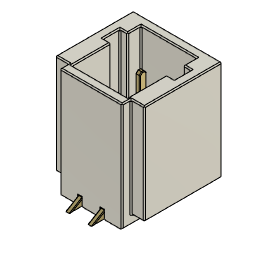
SH1.0mm_2P_立贴 (Autodesk Fusion 360 design; units mm, degrees)
Autodesk Fusion 360 part; units mm, degrees
sketch "草图1" plane through (0, 0, 0) normal (0, 0, 1) x (1, 0, 0) in component "Component'"
  line L0 (0, 0) -> (4, 0)
  line L1 (4, 0) -> (4, 3.9)
  line L2 (4, 3.9) -> (0, 3.9)
  line L3 (0, 3.9) -> (0, 0)
  dimension "d1" = 4
  dimension "d2" = 3.9
  constraint horizontal L0
  constraint vertical L1
  constraint horizontal L2
  constraint vertical L3
  constraint coincident L0.start L3.end
  measures "d1" distance of L0.start L0.end
  measures "d2" distance of L0.end L1.end
extrude "拉伸1" add sketch "草图1" along normal blind 4.9 makes body 1 in component "Component'"
sketch "草图2" plane through (0, 0, 4.9) normal (0, 0, 1) x (-1, 0, 0) in component "Component'"
  line L0 (0, -3.9) -> (0, 0)
  line L1 (0, 0) -> (-4, 0)
  line L2 (-4, 0) -> (-4, -3.9)
  line L3 (-4, -3.9) -> (0, -3.9)
  line L4 (-0.75, -0.4) -> (-3.25, -0.4)
  line L5 (-3.25, -0.4) -> (-3.25, -3.5)
  line L6 (-3.25, -3.5) -> (-0.75, -3.5)
  line L7 (-0.75, -3.5) -> (-0.75, -0.4)
  line L8 (-0.4, -2.9) -> (-3.6, -2.9)
  line L9 (-3.6, -2.9) -> (-3.6, -2.15)
  line L10 (-3.6, -2.15) -> (-0.4, -2.15)
  line L11 (-0.4, -2.15) -> (-0.4, -2.9)
  dimension "d5" = 2.5
  dimension "d6" = 0.75
  dimension "d7" = 0.4
  dimension "d8" = 0.4
  dimension "d9" = 3.2
  dimension "d10" = 0.4
  dimension "d11" = 1
  dimension "d12" = 0.75
  constraint horizontal L4
  constraint vertical L5
  constraint horizontal L6
  constraint vertical L7
  constraint horizontal L8
  constraint vertical L9
  constraint horizontal L10
  constraint vertical L11
  measures "d5" distance of L4.start L4.end
  measures "d6" distance of L2 L5
  measures "d7" distance of L3 L6
  measures "d8" distance of L1 L4
  measures "d9" distance of L9.end L10.end
  measures "d10" distance of L2 L9
  measures "d11" distance of L3 L8
  measures "d12" distance of L8.start L10.end
extrude "拉伸2" cut sketch "草图2" against normal blind 4 contours L4 L5 L7 L10 | L7 L8 L10 L11 | L5 L7 L8 L10 | L5 L8 L9 L10 | L5 L6 L7 L8 bodies 1 in component "Component'"
sketch "草图3" plane through (0, 0, 4.9) normal (0, 0, 1) x (-1, 0, 0) in component "Component'"
  line L0 (-3.25, -0.4) -> (-0.75, -0.4)
  line L1 (-0.75, -0.4) -> (-0.75, -2.15)
  line L2 (-0.75, -2.15) -> (-0.4, -2.15)
  line L3 (-0.4, -2.15) -> (-0.4, -2.9)
  line L4 (-0.4, -2.9) -> (-0.75, -2.9)
  line L5 (-0.75, -2.9) -> (-0.75, -3.5)
  line L6 (-0.75, -3.5) -> (-3.25, -3.5)
  line L7 (-3.25, -3.5) -> (-3.25, -2.9)
  line L8 (-3.25, -2.9) -> (-3.6, -2.9)
  line L9 (-3.6, -2.9) -> (-3.6, -2.15)
  line L10 (-3.6, -2.15) -> (-3.25, -2.15)
  line L11 (-3.25, -2.15) -> (-3.25, -0.4)
  line L12 (0, -3.9) -> (0, 0)
  line L13 (0, 0) -> (-4, 0)
  line L14 (-4, 0) -> (-4, -3.9)
  line L15 (-4, -3.9) -> (0, -3.9)
  line L16 (0, 0) -> (-0.6, 0)
  line L17 (-0.6, 0) -> (-0.6, -0.4)
  line L18 (-0.6, -0.4) -> (0, -0.4)
  line L19 (0, -0.4) -> (0, 0)
  line L20 (-4, 0) -> (-3.4, 0)
  line L21 (-3.4, 0) -> (-3.4, -0.4)
  line L22 (-3.4, -0.4) -> (-4, -0.4)
  line L23 (-4, -0.4) -> (-4, 0)
  dimension "d15" = 0.4
  dimension "d16" = 0.6
  dimension "d17" = 0.6
  dimension "d18" = 0.4
  constraint horizontal L16
  constraint vertical L17
  constraint horizontal L18
  constraint vertical L19
  constraint coincident L12.end L13.start
  constraint horizontal L20
  constraint vertical L21
  constraint horizontal L22
  constraint vertical L23
  constraint coincident L13.end L14.start
  measures "d15" distance of L16.end L17.end
  measures "d16" distance of L17.end L18.end
  measures "d17" distance of L21.end L22.end
  measures "d18" distance of L20.end L21.end
extrude "拉伸3" cut sketch "草图3" against normal up to surface (4.9 mm away) contours L12 L13 L16 L17 L18 L19 | L13 L14 L20 L21 L22 L23 bodies 1 in component "Component'"
sketch "草图4" plane through (0, 0, 0) normal (0, 0, -1) x (1, 0, 0) in component "Component'"
  line L0 (0.6, 0) -> (1.4, 0)
  line L1 (1.4, 0) -> (1.4, -3.9)
  line L2 (1.4, -3.9) -> (0.6, -3.9)
  line L3 (0.6, -3.9) -> (0.6, 0)
  line L4 (1.6, 0) -> (2.4, 0)
  line L5 (2.4, 0) -> (2.4, -3.9)
  line L6 (2.4, -3.9) -> (1.6, -3.9)
  line L7 (1.6, -3.9) -> (1.6, 0)
  line L8 (3.4, 0) -> (2.6, 0)
  line L9 (2.6, 0) -> (2.6, -3.9)
  line L10 (2.6, -3.9) -> (3.4, -3.9)
  line L11 (3.4, -3.9) -> (3.4, 0)
  line L12 (0, -3.9) -> (4, -3.9)
  line L13 (4, -3.9) -> (4, -3.5)
  line L14 (4, -3.5) -> (0, -3.5)
  line L15 (0, -3.5) -> (0, -3.9)
  line L16 (0, -3.5) -> (0, -0.4)
  line L17 (0, -0.4) -> (0.6, -0.4)
  line L18 (1.4, 0) -> (2.6, 0)
  line L19 (4, -3.5) -> (4, -0.4)
  line L20 (4, -0.4) -> (3.4, -0.4)
  point P0 (3.4, 0)
  dimension "d27" = 0.8
  dimension "d28" = 0.2
  dimension "d29" = 0.2
  dimension "d30" = 0.8
  dimension "d31" = 0.8
  dimension "d32" = 0.4
  constraint horizontal L0
  constraint vertical L1
  constraint horizontal L2
  constraint vertical L3
  constraint horizontal L4
  constraint vertical L5
  constraint horizontal L6
  constraint vertical L7
  constraint horizontal L8
  constraint vertical L9
  constraint horizontal L10
  constraint vertical L11
  constraint coincident P0 L8.start
  constraint horizontal L12
  constraint vertical L13
  constraint horizontal L14
  constraint vertical L15
  constraint perpendicular L14 L16
  constraint coincident L3 L17.end
  constraint perpendicular L3 L17
  constraint perpendicular L9 L18
  constraint perpendicular L14 L19
  constraint coincident L11 L20.end
  constraint perpendicular L11 L20
  measures "d27" distance of L4.start L4.end
  measures "d28" distance of L5 L9
  measures "d29" distance of L1 L7
  measures "d30" distance of P0 L8.end
  measures "d31" distance of L0.start L0.end
  measures "d32" distance of L12.end L13.end
extrude "拉伸5" cut sketch "草图4" against normal blind 0.4 contours L1 L7 L14 L18 | L3 L14 L16 L17 | L1 L7 L12 L14 | L1 L2 L3 L12 L14 | L3 L12 L14 L15 | L5 L6 L7 L12 L14 | L5 L9 L14 L18 | L5 L9 L12 L14 | L9 L10 L11 L12 L14 | L11 L12 L13 L14 | L11 L14 L19 L20 bodies 1 in component "Component'"
sketch "草图6" plane through (0, 0, 0.4) normal (0, 0, -1) x (1, 0, 0) in component "Component'"
  line L0 (0, -0.4) -> (0, -3.9)
  line L1 (0, -3.9) -> (4, -3.9)
  line L2 (4, -3.9) -> (4, -0.4)
  line L3 (4, -0.4) -> (3.4, -0.4)
  line L4 (3.4, -0.4) -> (3.4, -3.5)
  line L5 (3.4, -3.5) -> (2.6, -3.5)
  line L6 (2.6, -3.5) -> (2.6, 0)
  line L7 (2.6, 0) -> (2.4, 0)
  line L8 (2.4, 0) -> (2.4, -3.5)
  line L9 (2.4, -3.5) -> (1.6, -3.5)
  line L10 (1.6, -3.5) -> (1.6, 0)
  line L11 (1.6, 0) -> (1.4, 0)
  line L12 (1.4, 0) -> (1.4, -3.5)
  line L13 (1.4, -3.5) -> (0.6, -3.5)
  line L14 (0.6, -3.5) -> (0.6, -0.4)
  line L15 (0.6, -0.4) -> (0, -0.4)
  line L16 (1.4, -2.6) -> (1.6, -2.6)
  line L17 (1.6, -2.6) -> (1.6, -2.9)
  line L18 (1.6, -2.9) -> (1.4, -2.9)
  line L19 (1.4, -2.9) -> (1.4, -2.6)
  line L20 (2.4, -2.6) -> (2.6, -2.6)
  line L21 (2.6, -2.6) -> (2.6, -2.9)
  line L22 (2.6, -2.9) -> (2.4, -2.9)
  line L23 (2.4, -2.9) -> (2.4, -2.6)
  dimension "d35" = 0.3
  dimension "d36" = 1
  constraint horizontal L16
  constraint vertical L17
  constraint horizontal L18
  constraint vertical L19
  constraint coincident L10 L17.end
  constraint coincident L12 L16.start
  constraint horizontal L20
  constraint vertical L21
  constraint horizontal L22
  constraint vertical L23
  constraint coincident L6 L21.end
  constraint coincident L8 L20.start
  constraint collinear L18 L22
  constraint collinear L16 L20
  measures "d35" distance of L16.start L18.end
  measures "d36" distance of L1 L18
extrude "拉伸6" cut sketch "草图6" against normal up to surface (0.5 mm away) contours L10 L12 L16 L17 L18 L19 | L6 L8 L20 L21 L22 L23 bodies 1 in component "Component'"
sketch "草图1 (2)" plane through (1.4, 0, 0) normal (1, 0, 0) x (0, 1, 0) in component "Component''"
  line L0 (0, 0) -> (3.5, 0)
  line L1 (3.5, 0) -> (3.5, 0.4)
  line L2 (3.5, 0.4) -> (2.9, 0.4)
  line L3 (2.9, 0.4) -> (2.9, 0.9)
  line L4 (2.9, 0.9) -> (2.6, 0.9)
  line L5 (2.6, 0.9) -> (2.6, 0.4)
  line L6 (2.6, 0.4) -> (0, 0.4)
  line L7 (0, 0.4) -> (0, 0)
  line L8 (2.9, 0.4) -> (2.9, 3.9)
  line L9 (2.9, 3.9) -> (2.6, 3.9)
  line L10 (2.6, 3.9) -> (2.6, 0.4)
  line L11 (0.398, 0.4) -> (0.0284, 0.3471)
  line L12 (0.0284, 0.3471) -> (-0.55, 0)
  line L13 (-0.55, 0) -> (2.9, 0)
  line L14 (2.9, 0.4) -> (2.9, 0)
  line L15 (0, 0) -> (0, 4.9)
  dimension "d39" = 3.5
  dimension "d41" = 0.55
  constraint coincident L2.end L3.start
  constraint perpendicular L4 L8
  constraint perpendicular L8 L9
  constraint coincident L5.end L6.start
  constraint coincident L6 L11.start
  constraint coincident L0 L13.end
  constraint perpendicular L7 L13
  constraint vertical L14
  measures "d39" distance of L2.end L8.end
  measures "d41" distance of L12.end L15
extrude "拉伸1'" add sketch "草图1 (2)" along normal blind 0.2 separate body contours L0 L3 L4 L5 L6 L7 L8 L10 L11 L12 L13 L14 L15 | L7 L12 L13 L15 | L4 L8 L9 L10 makes body 2 in component "Component''"
chamfer "倒角1" distance 0.1 angle 45 2 edges at (1.5, 2.6, 3.9) (1.5, 2.9, 3.9) on bodies 2 in component "Component''"
fillet "圆角1" radius 0.25 1 edges at (1.5, 2.9, 0) on bodies 2 in component "Component''"
fillet "圆角2" radius 0.03 2 faces at (1.6, 0.8327, 0.1333) (1.4, 0.8327, 0.1333) on bodies 2 in component "Component''"
pattern_linear "R-阵列1" count 2 spacing 1 along (1, 0, 0) of bodies 2 makes body 3 in component "Component''"
chamfer "倒角1'" distance 0.05 angle 45 1 faces at (0.3333, 0.9833, 4.9) on bodies 1 in component "Component'"
chamfer "倒角2" distance 0.05 angle 45 31 edges at (0, 3.9, 2.625) (0, 0.4, 2.625) (0.6, 0.4, 2.625) (0.6, 0, 2.425) (3.4, 0, 2.425) (3.4, 0.4, 2.625) (4, 0.4, 2.625) (4, 3.9, 2.625) (0.75, 0.4, 2.875) (3.25, 0.4, 2.875) (3.25, 3.5, 2.875) (3.6, 2.9, 2.875) (3.6, 2.15, 2.875) (3.25, 2.9, 2.875) (3.25, 2.15, 2.875) (0.75, 2.15, 2.875) (0.4, 2.15, 2.875) (0.4, 2.9, 2.875) (0.75, 2.9, 2.875) (0.75, 3.5, 2.875) (0.6, 1.75, 0) (1.4, 1.75, 0) (1.6, 1.75, 0) (2.4, 1.75, 0) (2.6, 1.75, 0) (3.4, 1.75, 0) (0, 2.15, 0.4) (4, 2.15, 0.4) (3.7, 0.4, 0.4) (0.3, 0.4, 0.4) (2, 3.9, 0.4) on bodies 1 in component "Component'"
component "Component'" placed x (1, 0, 0) y (0, 1, 0) z (0, 0, 1) at (0, 0, 0)
component "Component''" placed x (1, 0, 0) y (0, 1, 0) z (0, 0, 1) at (0, 0, 0)
equation "d17 = d16"
equation "d18 = d15"
